Autodesk Inventor part; units mm, degrees
(part 2 of 6)
  line L875 (-91.9006, -60.9474) -> (-91.9173, -60.9168) projected
  line L876 (-91.9173, -60.9168) -> (-91.9334, -60.8858) projected
  line L877 (-91.9334, -60.8858) -> (-91.949, -60.8546) projected
  line L878 (-91.949, -60.8546) -> (-91.964, -60.823) projected
  line L879 (-91.964, -60.823) -> (-91.9785, -60.7913) projected
  line L880 (-91.9785, -60.7913) -> (-91.9924, -60.7593) projected
  line L881 (-91.9924, -60.7593) -> (-92.0058, -60.727) projected
  line L882 (-92.0058, -60.727) -> (-92.0186, -60.6945) projected
  line L883 (-92.0186, -60.6945) -> (-92.0308, -60.6618) projected
  line L884 (-92.0308, -60.6618) -> (-92.0424, -60.6289) projected
  line L885 (-92.0424, -60.6289) -> (-92.0535, -60.5958) projected
  line L886 (-92.0535, -60.5958) -> (-92.064, -60.5626) projected
  line L887 (-92.064, -60.5626) -> (-92.0739, -60.5291) projected
  line L888 (-92.0739, -60.5291) -> (-92.0833, -60.4954) projected
  line L889 (-92.0833, -60.4954) -> (-92.092, -60.4617) projected
  line L890 (-92.092, -60.4617) -> (-92.1001, -60.4277) projected
  line L891 (-92.1001, -60.4277) -> (-92.1077, -60.3936) projected
  line L892 (-92.1077, -60.3936) -> (-92.1147, -60.3594) projected
  line L893 (-92.1147, -60.3594) -> (-92.121, -60.3251) projected
  line L894 (-92.121, -60.3251) -> (-92.1268, -60.2907) projected
  line L895 (-92.1268, -60.2907) -> (-92.1319, -60.2562) projected
  line L896 (-92.1319, -60.2562) -> (-92.1365, -60.2215) projected
  line L897 (-92.1365, -60.2215) -> (-92.1404, -60.1869) projected
  line L898 (-92.1404, -60.1869) -> (-92.1438, -60.1521) projected
  line L899 (-92.1438, -60.1521) -> (-92.1465, -60.1173) projected
  line L900 (-92.1465, -60.1173) -> (-92.1487, -60.0825) projected
  line L901 (-92.1487, -60.0825) -> (-92.1502, -60.0476) projected
  line L902 (-92.1502, -60.0476) -> (-92.1511, -60.0127) projected
  line L903 (-92.1511, -60.0127) -> (-92.1514, -59.9778) projected
  line L904 (-92.1514, -59.9778) -> (-92.1511, -59.9429) projected
  line L905 (-92.1511, -59.9429) -> (-92.1502, -59.908) projected
  line L906 (-92.1502, -59.908) -> (-92.1487, -59.8731) projected
  line L907 (-92.1487, -59.8731) -> (-92.1465, -59.8383) projected
  line L908 (-92.1465, -59.8383) -> (-92.1438, -59.8035) projected
  line L909 (-92.1438, -59.8035) -> (-92.1404, -59.7688) projected
  line L910 (-92.1404, -59.7688) -> (-92.1365, -59.7341) projected
  line L911 (-92.1365, -59.7341) -> (-92.1319, -59.6995) projected
  line L912 (-92.1319, -59.6995) -> (-92.1268, -59.6649) projected
  line L913 (-92.1268, -59.6649) -> (-92.121, -59.6305) projected
  line L914 (-92.121, -59.6305) -> (-92.1147, -59.5962) projected
  line L915 (-92.1147, -59.5962) -> (-92.1077, -59.562) projected
  line L916 (-92.1077, -59.562) -> (-92.1001, -59.5279) projected
  line L917 (-92.1001, -59.5279) -> (-92.092, -59.494) projected
  line L918 (-92.092, -59.494) -> (-92.0833, -59.4602) projected
  line L919 (-92.0833, -59.4602) -> (-92.0739, -59.4265) projected
  line L920 (-92.0739, -59.4265) -> (-92.064, -59.3931) projected
  line L921 (-92.064, -59.3931) -> (-92.0535, -59.3598) projected
  line L922 (-92.0535, -59.3598) -> (-92.0424, -59.3267) projected
  line L923 (-92.0424, -59.3267) -> (-92.0308, -59.2938) projected
  line L924 (-92.0308, -59.2938) -> (-92.0186, -59.2611) projected
  line L925 (-92.0186, -59.2611) -> (-92.0058, -59.2286) projected
  line L926 (-92.0058, -59.2286) -> (-91.9924, -59.1963) projected
  line L927 (-91.9924, -59.1963) -> (-91.9785, -59.1643) projected
  line L928 (-91.9785, -59.1643) -> (-91.964, -59.1326) projected
  line L929 (-91.964, -59.1326) -> (-91.949, -59.1011) projected
  line L930 (-91.949, -59.1011) -> (-91.9334, -59.0698) projected
  line L931 (-91.9334, -59.0698) -> (-91.9173, -59.0389) projected
  line L932 (-91.9173, -59.0389) -> (-91.9006, -59.0082) projected
  line L933 (-91.9006, -59.0082) -> (-91.8835, -58.9778) projected
  line L934 (-91.8835, -58.9778) -> (-91.8657, -58.9477) projected
  line L935 (-91.8657, -58.9477) -> (-91.8475, -58.918) projected
  line L936 (-91.8475, -58.918) -> (-91.8287, -58.8885) projected
  line L937 (-91.8287, -58.8885) -> (-91.8095, -58.8594) projected
  line L938 (-91.8095, -58.8594) -> (-91.7897, -58.8307) projected
  line L939 (-91.7897, -58.8307) -> (-91.7694, -58.8022) projected
  line L940 (-91.7694, -58.8022) -> (-91.7487, -58.7742) projected
  line L941 (-91.7487, -58.7742) -> (-91.7274, -58.7465) projected
  line L942 (-91.7274, -58.7465) -> (-91.7057, -58.7192) projected
  line L943 (-91.7057, -58.7192) -> (-91.6835, -58.6922) projected
  line L944 (-91.6835, -58.6922) -> (-91.6608, -58.6657) projected
  line L945 (-91.6608, -58.6657) -> (-91.6377, -58.6396) projected
  line L946 (-91.6377, -58.6396) -> (-91.6141, -58.6138) projected
  line L947 (-91.6141, -58.6138) -> (-91.5901, -58.5885) projected
  line L948 (-91.5901, -58.5885) -> (-91.5656, -58.5636) projected
  line L949 (-91.5656, -58.5636) -> (-91.5407, -58.5391) projected
  line L950 (-91.5407, -58.5391) -> (-91.5154, -58.5151) projected
  line L951 (-91.5154, -58.5151) -> (-91.4897, -58.4915) projected
  line L952 (-91.4897, -58.4915) -> (-91.4635, -58.4684) projected
  line L953 (-91.4635, -58.4684) -> (-91.437, -58.4457) projected
  line L954 (-91.437, -58.4457) -> (-91.41, -58.4235) projected
  line L955 (-91.41, -58.4235) -> (-91.3827, -58.4018) projected
  line L956 (-91.3827, -58.4018) -> (-91.355, -58.3805) projected
  line L957 (-91.355, -58.3805) -> (-91.327, -58.3598) projected
  line L958 (-91.327, -58.3598) -> (-91.2986, -58.3395) projected
  line L959 (-91.2986, -58.3395) -> (-91.2698, -58.3197) projected
  line L960 (-91.2698, -58.3197) -> (-91.2407, -58.3005) projected
  line L961 (-91.2407, -58.3005) -> (-91.2112, -58.2817) projected
  line L962 (-91.2112, -58.2817) -> (-91.1815, -58.2635) projected
  line L963 (-91.1815, -58.2635) -> (-91.1514, -58.2458) projected
  line L964 (-91.1514, -58.2458) -> (-91.121, -58.2286) projected
  line L965 (-91.121, -58.2286) -> (-91.0904, -58.2119) projected
  line L966 (-91.0904, -58.2119) -> (-91.0594, -58.1958) projected
  line L967 (-91.0594, -58.1958) -> (-91.0282, -58.1802) projected
  line L968 (-91.0282, -58.1802) -> (-90.9966, -58.1652) projected
  line L969 (-90.9966, -58.1652) -> (-90.9649, -58.1507) projected
  line L970 (-90.9649, -58.1507) -> (-90.9329, -58.1368) projected
  line L971 (-90.9329, -58.1368) -> (-90.9006, -58.1234) projected
  line L972 (-90.9006, -58.1234) -> (-90.8681, -58.1107) projected
  line L973 (-90.8681, -58.1107) -> (-90.8354, -58.0984) projected
  line L974 (-90.8354, -58.0984) -> (-90.8025, -58.0868) projected
  line L975 (-90.8025, -58.0868) -> (-90.7694, -58.0757) projected
  line L976 (-90.7694, -58.0757) -> (-90.7362, -58.0652) projected
  line L977 (-90.7362, -58.0652) -> (-90.7027, -58.0553) projected
  line L978 (-90.7027, -58.0553) -> (-90.669, -58.046) projected
  line L979 (-90.669, -58.046) -> (-90.6353, -58.0372) projected
  line L980 (-90.6353, -58.0372) -> (-90.6013, -58.0291) projected
  line L981 (-90.6013, -58.0291) -> (-90.5672, -58.0215) projected
  line L982 (-90.5672, -58.0215) -> (-90.533, -58.0146) projected
  line L983 (-90.533, -58.0146) -> (-90.4987, -58.0082) projected
  line L984 (-90.4987, -58.0082) -> (-90.4643, -58.0024) projected
  line L985 (-90.4643, -58.0024) -> (-90.4298, -57.9973) projected
  line L986 (-90.4298, -57.9973) -> (-90.3951, -57.9927) projected
  line L987 (-90.3951, -57.9927) -> (-90.3605, -57.9888) projected
  line L988 (-90.3605, -57.9888) -> (-90.3257, -57.9854) projected
  line L989 (-90.3257, -57.9854) -> (-90.2909, -57.9827) projected
  line L990 (-90.2909, -57.9827) -> (-90.2561, -57.9806) projected
  line L991 (-90.2561, -57.9806) -> (-90.2212, -57.979) projected
  line L992 (-90.2212, -57.979) -> (-90.1863, -57.9781) projected
  line L993 (-90.1863, -57.9781) -> (-90.1514, -57.9778) projected
  line L994 (-90.1514, -57.9778) -> (-90.1165, -57.9781) projected
  line L995 (-90.1165, -57.9781) -> (-90.0816, -57.979) projected
  line L996 (-90.0816, -57.979) -> (-90.0467, -57.9806) projected
  line L997 (-90.0467, -57.9806) -> (-90.0119, -57.9827) projected
  line L998 (-90.0119, -57.9827) -> (-89.9771, -57.9854) projected
  line L999 (-89.9771, -57.9854) -> (-89.9424, -57.9888) projected
  line L1000 (-89.9424, -57.9888) -> (-89.9077, -57.9927) projected
  line L1001 (-89.9077, -57.9927) -> (-89.8731, -57.9973) projected
  line L1002 (-89.8731, -57.9973) -> (-89.8385, -58.0024) projected
  line L1003 (-89.8385, -58.0024) -> (-89.8041, -58.0082) projected
  line L1004 (-89.8041, -58.0082) -> (-89.7698, -58.0146) projected
  line L1005 (-89.7698, -58.0146) -> (-89.7356, -58.0215) projected
  line L1006 (-89.7356, -58.0215) -> (-89.7015, -58.0291) projected
  line L1007 (-89.7015, -58.0291) -> (-89.6676, -58.0372) projected
  line L1008 (-89.6676, -58.0372) -> (-89.6338, -58.046) projected
  line L1009 (-89.6338, -58.046) -> (-89.6001, -58.0553) projected
  line L1010 (-89.6001, -58.0553) -> (-89.5667, -58.0652) projected
  line L1011 (-89.5667, -58.0652) -> (-89.5334, -58.0757) projected
  line L1012 (-89.5334, -58.0757) -> (-89.5003, -58.0868) projected
  line L1013 (-89.5003, -58.0868) -> (-89.4674, -58.0984) projected
  line L1014 (-89.4674, -58.0984) -> (-89.4347, -58.1107) projected
  line L1015 (-89.4347, -58.1107) -> (-89.4022, -58.1234) projected
  line L1016 (-89.4022, -58.1234) -> (-89.3699, -58.1368) projected
  line L1017 (-89.3699, -58.1368) -> (-89.3379, -58.1507) projected
  line L1018 (-89.3379, -58.1507) -> (-89.3062, -58.1652) projected
  line L1019 (-89.3062, -58.1652) -> (-89.2747, -58.1802) projected
  line L1020 (-89.2747, -58.1802) -> (-89.2434, -58.1958) projected
  line L1021 (-89.2434, -58.1958) -> (-89.2125, -58.2119) projected
  line L1022 (-89.2125, -58.2119) -> (-89.1818, -58.2286) projected
  line L1023 (-89.1818, -58.2286) -> (-89.1514, -58.2458) projected
  line L1024 (-89.1514, -58.2458) -> (-89.1213, -58.2635) projected
  line L1025 (-89.1213, -58.2635) -> (-89.0916, -58.2817) projected
  line L1026 (-89.0916, -58.2817) -> (-89.0621, -58.3005) projected
  line L1027 (-89.0621, -58.3005) -> (-89.033, -58.3197) projected
  line L1028 (-89.033, -58.3197) -> (-89.0043, -58.3395) projected
  line L1029 (-89.0043, -58.3395) -> (-88.9758, -58.3598) projected
  line L1030 (-88.9758, -58.3598) -> (-88.9478, -58.3805) projected
  line L1031 (-88.9478, -58.3805) -> (-88.9201, -58.4018) projected
  line L1032 (-88.9201, -58.4018) -> (-88.8928, -58.4235) projected
  line L1033 (-88.8928, -58.4235) -> (-88.8658, -58.4457) projected
  line L1034 (-88.8658, -58.4457) -> (-88.8393, -58.4684) projected
  line L1035 (-88.8393, -58.4684) -> (-88.8132, -58.4915) projected
  line L1036 (-88.8132, -58.4915) -> (-88.7874, -58.5151) projected
  line L1037 (-88.7874, -58.5151) -> (-88.7621, -58.5391) projected
  line L1038 (-88.7621, -58.5391) -> (-88.7372, -58.5636) projected
  line L1039 (-88.7372, -58.5636) -> (-88.7127, -58.5885) projected
  line L1040 (-88.7127, -58.5885) -> (-88.6887, -58.6138) projected
  line L1041 (-88.6887, -58.6138) -> (-88.6651, -58.6396) projected
  line L1042 (-88.6651, -58.6396) -> (-88.642, -58.6657) projected
  line L1043 (-88.642, -58.6657) -> (-88.6193, -58.6922) projected
  line L1044 (-88.6193, -58.6922) -> (-88.5971, -58.7192) projected
  line L1045 (-88.5971, -58.7192) -> (-88.5754, -58.7465) projected
  line L1046 (-88.5754, -58.7465) -> (-88.5541, -58.7742) projected
  line L1047 (-88.5541, -58.7742) -> (-88.5334, -58.8022) projected
  line L1048 (-88.5334, -58.8022) -> (-88.5131, -58.8307) projected
  line L1049 (-88.5131, -58.8307) -> (-88.4933, -58.8594) projected
  line L1050 (-88.4933, -58.8594) -> (-88.4741, -58.8885) projected
  line L1051 (-88.4741, -58.8885) -> (-88.4553, -58.918) projected
  line L1052 (-88.4553, -58.918) -> (-88.4371, -58.9477) projected
  line L1053 (-88.4371, -58.9477) -> (-88.4194, -58.9778) projected
  line L1054 (-88.4194, -58.9778) -> (-88.4022, -59.0082) projected
  line L1055 (-88.4022, -59.0082) -> (-88.3855, -59.0389) projected
  line L1056 (-88.3855, -59.0389) -> (-88.3694, -59.0698) projected
  line L1057 (-88.3694, -59.0698) -> (-88.3538, -59.1011) projected
  line L1058 (-88.3538, -59.1011) -> (-88.3388, -59.1326) projected
  line L1059 (-88.3388, -59.1326) -> (-88.3243, -59.1643) projected
  line L1060 (-88.3243, -59.1643) -> (-88.3104, -59.1963) projected
  line L1061 (-88.3104, -59.1963) -> (-88.297, -59.2286) projected
  line L1062 (-88.297, -59.2286) -> (-88.2843, -59.2611) projected
  line L1063 (-88.2843, -59.2611) -> (-88.272, -59.2938) projected
  line L1064 (-88.272, -59.2938) -> (-88.2604, -59.3267) projected
  line L1065 (-88.2604, -59.3267) -> (-88.2493, -59.3598) projected
  line L1066 (-88.2493, -59.3598) -> (-88.2388, -59.3931) projected
  line L1067 (-88.2388, -59.3931) -> (-88.2289, -59.4265) projected
  line L1068 (-88.2289, -59.4265) -> (-88.2196, -59.4602) projected
  line L1069 (-88.2196, -59.4602) -> (-88.2108, -59.494) projected
  line L1070 (-88.2108, -59.494) -> (-88.2027, -59.5279) projected
  line L1071 (-88.2027, -59.5279) -> (-88.1951, -59.562) projected
  line L1072 (-88.1951, -59.562) -> (-88.1882, -59.5962) projected
  line L1073 (-88.1882, -59.5962) -> (-88.1818, -59.6305) projected
  line L1074 (-88.1818, -59.6305) -> (-88.176, -59.6649) projected
  line L1075 (-88.176, -59.6649) -> (-88.1709, -59.6995) projected
  line L1076 (-88.1709, -59.6995) -> (-88.1663, -59.7341) projected
  line L1077 (-88.1663, -59.7341) -> (-88.1624, -59.7688) projected
  line L1078 (-88.1624, -59.7688) -> (-88.159, -59.8035) projected
  line L1079 (-88.159, -59.8035) -> (-88.1563, -59.8383) projected
  line L1080 (-88.1563, -59.8383) -> (-88.1542, -59.8731) projected
  line L1081 (-88.1542, -59.8731) -> (-88.1526, -59.908) projected
  line L1082 (-88.1526, -59.908) -> (-88.1517, -59.9429) projected
  line L1083 (-88.1517, -59.9429) -> (-88.1514, -59.9778) projected
  line L1084 (-88.1563, 60.1617) -> (-88.1542, 60.1269) projected
  line L1085 (-88.1542, 60.1269) -> (-88.1526, 60.092) projected
  line L1086 (-88.1526, 60.092) -> (-88.1517, 60.0571) projected
  line L1087 (-88.1517, 60.0571) -> (-88.1514, 60.0222) projected
  line L1088 (-88.1514, 60.0222) -> (-88.1517, 59.9873) projected
  line L1089 (-88.1517, 59.9873) -> (-88.1526, 59.9524) projected
  line L1090 (-88.1526, 59.9524) -> (-88.1542, 59.9175) projected
  line L1091 (-88.1542, 59.9175) -> (-88.1563, 59.8827) projected
  line L1092 (-88.1563, 59.8827) -> (-88.159, 59.8479) projected
  line L1093 (-88.159, 59.8479) -> (-88.1624, 59.8131) projected
  line L1094 (-88.1624, 59.8131) -> (-88.1663, 59.7785) projected
  line L1095 (-88.1663, 59.7785) -> (-88.1709, 59.7439) projected
  line L1096 (-88.1709, 59.7439) -> (-88.176, 59.7093) projected
  line L1097 (-88.176, 59.7093) -> (-88.1818, 59.6749) projected
  line L1098 (-88.1818, 59.6749) -> (-88.1882, 59.6406) projected
  line L1099 (-88.1882, 59.6406) -> (-88.1951, 59.6064) projected
  line L1100 (-88.1951, 59.6064) -> (-88.2027, 59.5723) projected
  line L1101 (-88.2027, 59.5723) -> (-88.2108, 59.5384) projected
  line L1102 (-88.2108, 59.5384) -> (-88.2196, 59.5046) projected
  line L1103 (-88.2196, 59.5046) -> (-88.2289, 59.4709) projected
  line L1104 (-88.2289, 59.4709) -> (-88.2388, 59.4375) projected
  line L1105 (-88.2388, 59.4375) -> (-88.2493, 59.4042) projected
  line L1106 (-88.2493, 59.4042) -> (-88.2604, 59.3711) projected
  line L1107 (-88.2604, 59.3711) -> (-88.272, 59.3382) projected
  line L1108 (-88.272, 59.3382) -> (-88.2843, 59.3055) projected
  line L1109 (-88.2843, 59.3055) -> (-88.297, 59.273) projected
  line L1110 (-88.297, 59.273) -> (-88.3104, 59.2407) projected
  line L1111 (-88.3104, 59.2407) -> (-88.3243, 59.2087) projected
  line L1112 (-88.3243, 59.2087) -> (-88.3388, 59.177) projected
  line L1113 (-88.3388, 59.177) -> (-88.3538, 59.1455) projected
  line L1114 (-88.3538, 59.1455) -> (-88.3694, 59.1142) projected
  line L1115 (-88.3694, 59.1142) -> (-88.3855, 59.0833) projected
  line L1116 (-88.3855, 59.0833) -> (-88.4022, 59.0526) projected
  line L1117 (-88.4022, 59.0526) -> (-88.4194, 59.0222) projected
  line L1118 (-88.4194, 59.0222) -> (-88.4371, 58.9921) projected
  line L1119 (-88.4371, 58.9921) -> (-88.4553, 58.9624) projected
  line L1120 (-88.4553, 58.9624) -> (-88.4741, 58.9329) projected
  line L1121 (-88.4741, 58.9329) -> (-88.4933, 58.9038) projected
  line L1122 (-88.4933, 58.9038) -> (-88.5131, 58.8751) projected
  line L1123 (-88.5131, 58.8751) -> (-88.5334, 58.8466) projected
  line L1124 (-88.5334, 58.8466) -> (-88.5541, 58.8186) projected
  line L1125 (-88.5541, 58.8186) -> (-88.5754, 58.7909) projected
  line L1126 (-88.5754, 58.7909) -> (-88.5971, 58.7636) projected
  line L1127 (-88.5971, 58.7636) -> (-88.6193, 58.7366) projected
  line L1128 (-88.6193, 58.7366) -> (-88.642, 58.7101) projected
  line L1129 (-88.642, 58.7101) -> (-88.6651, 58.6839) projected
  line L1130 (-88.6651, 58.6839) -> (-88.6887, 58.6582) projected
  line L1131 (-88.6887, 58.6582) -> (-88.7127, 58.6329) projected
  line L1132 (-88.7127, 58.6329) -> (-88.7372, 58.608) projected
  line L1133 (-88.7372, 58.608) -> (-88.7621, 58.5835) projected
  line L1134 (-88.7621, 58.5835) -> (-88.7874, 58.5595) projected
  line L1135 (-88.7874, 58.5595) -> (-88.8132, 58.5359) projected
  line L1136 (-88.8132, 58.5359) -> (-88.8393, 58.5128) projected
  line L1137 (-88.8393, 58.5128) -> (-88.8658, 58.4901) projected
  line L1138 (-88.8658, 58.4901) -> (-88.8928, 58.4679) projected
  line L1139 (-88.8928, 58.4679) -> (-88.9201, 58.4462) projected
  line L1140 (-88.9201, 58.4462) -> (-88.9478, 58.4249) projected
  line L1141 (-88.9478, 58.4249) -> (-88.9758, 58.4042) projected
  line L1142 (-88.9758, 58.4042) -> (-89.0043, 58.3839) projected
  line L1143 (-89.0043, 58.3839) -> (-89.033, 58.3641) projected
  line L1144 (-89.033, 58.3641) -> (-89.0621, 58.3449) projected
  line L1145 (-89.0621, 58.3449) -> (-89.0916, 58.3261) projected
  line L1146 (-89.0916, 58.3261) -> (-89.1213, 58.3079) projected
  line L1147 (-89.1213, 58.3079) -> (-89.1514, 58.2902) projected
  line L1148 (-89.1514, 58.2902) -> (-89.1818, 58.273) projected
  line L1149 (-89.1818, 58.273) -> (-89.2125, 58.2563) projected
  line L1150 (-89.2125, 58.2563) -> (-89.2434, 58.2402) projected
  line L1151 (-89.2434, 58.2402) -> (-89.2747, 58.2246) projected
  line L1152 (-89.2747, 58.2246) -> (-89.3062, 58.2096) projected
  line L1153 (-89.3062, 58.2096) -> (-89.3379, 58.1951) projected
  line L1154 (-89.3379, 58.1951) -> (-89.3699, 58.1812) projected
  line L1155 (-89.3699, 58.1812) -> (-89.4022, 58.1678) projected
  line L1156 (-89.4022, 58.1678) -> (-89.4347, 58.155) projected
  line L1157 (-89.4347, 58.155) -> (-89.4674, 58.1428) projected
  line L1158 (-89.4674, 58.1428) -> (-89.5003, 58.1312) projected
  line L1159 (-89.5003, 58.1312) -> (-89.5334, 58.1201) projected
  line L1160 (-89.5334, 58.1201) -> (-89.5667, 58.1096) projected
  line L1161 (-89.5667, 58.1096) -> (-89.6001, 58.0997) projected
  line L1162 (-89.6001, 58.0997) -> (-89.6338, 58.0904) projected
  line L1163 (-89.6338, 58.0904) -> (-89.6676, 58.0816) projected
  line L1164 (-89.6676, 58.0816) -> (-89.7015, 58.0735) projected
  line L1165 (-89.7015, 58.0735) -> (-89.7356, 58.0659) projected
  line L1166 (-89.7356, 58.0659) -> (-89.7698, 58.059) projected
  line L1167 (-89.7698, 58.059) -> (-89.8041, 58.0526) projected
  line L1168 (-89.8041, 58.0526) -> (-89.8385, 58.0468) projected
  line L1169 (-89.8385, 58.0468) -> (-89.8731, 58.0417) projected
  line L1170 (-89.8731, 58.0417) -> (-89.9077, 58.0371) projected
  line L1171 (-89.9077, 58.0371) -> (-89.9424, 58.0332) projected
  line L1172 (-89.9424, 58.0332) -> (-89.9771, 58.0298) projected
  line L1173 (-89.9771, 58.0298) -> (-90.0119, 58.0271) projected
  line L1174 (-90.0119, 58.0271) -> (-90.0467, 58.0249) projected
  line L1175 (-90.0467, 58.0249) -> (-90.0816, 58.0234) projected
  line L1176 (-90.0816, 58.0234) -> (-90.1165, 58.0225) projected
  line L1177 (-90.1165, 58.0225) -> (-90.1514, 58.0222) projected
  line L1178 (-90.1514, 58.0222) -> (-90.1863, 58.0225) projected
  line L1179 (-90.1863, 58.0225) -> (-90.2212, 58.0234) projected
  line L1180 (-90.2212, 58.0234) -> (-90.2561, 58.0249) projected
  line L1181 (-90.2561, 58.0249) -> (-90.2909, 58.0271) projected
  line L1182 (-90.2909, 58.0271) -> (-90.3257, 58.0298) projected
  line L1183 (-90.3257, 58.0298) -> (-90.3605, 58.0332) projected
  line L1184 (-90.3605, 58.0332) -> (-90.3951, 58.0371) projected
  line L1185 (-90.3951, 58.0371) -> (-90.4298, 58.0417) projected
  line L1186 (-90.4298, 58.0417) -> (-90.4643, 58.0468) projected
  line L1187 (-90.4643, 58.0468) -> (-90.4987, 58.0526) projected
  line L1188 (-90.4987, 58.0526) -> (-90.533, 58.059) projected
  line L1189 (-90.533, 58.059) -> (-90.5672, 58.0659) projected
  line L1190 (-90.5672, 58.0659) -> (-90.6013, 58.0735) projected
  line L1191 (-90.6013, 58.0735) -> (-90.6353, 58.0816) projected
  line L1192 (-90.6353, 58.0816) -> (-90.669, 58.0904) projected
  line L1193 (-90.669, 58.0904) -> (-90.7027, 58.0997) projected
  line L1194 (-90.7027, 58.0997) -> (-90.7362, 58.1096) projected
  line L1195 (-90.7362, 58.1096) -> (-90.7694, 58.1201) projected
  line L1196 (-90.7694, 58.1201) -> (-90.8025, 58.1312) projected
  line L1197 (-90.8025, 58.1312) -> (-90.8354, 58.1428) projected
  line L1198 (-90.8354, 58.1428) -> (-90.8681, 58.155) projected
  line L1199 (-90.8681, 58.155) -> (-90.9006, 58.1678) projected
  line L1200 (-90.9006, 58.1678) -> (-90.9329, 58.1812) projected
  line L1201 (-90.9329, 58.1812) -> (-90.9649, 58.1951) projected
  line L1202 (-90.9649, 58.1951) -> (-90.9966, 58.2096) projected
  line L1203 (-90.9966, 58.2096) -> (-91.0282, 58.2246) projected
  line L1204 (-91.0282, 58.2246) -> (-91.0594, 58.2402) projected
  line L1205 (-91.0594, 58.2402) -> (-91.0904, 58.2563) projected
  line L1206 (-91.0904, 58.2563) -> (-91.121, 58.273) projected
  line L1207 (-91.121, 58.273) -> (-91.1514, 58.2902) projected
  line L1208 (-91.1514, 58.2902) -> (-91.1815, 58.3079) projected
  line L1209 (-91.1815, 58.3079) -> (-91.2112, 58.3261) projected
  line L1210 (-91.2112, 58.3261) -> (-91.2407, 58.3449) projected
  line L1211 (-91.2407, 58.3449) -> (-91.2698, 58.3641) projected
  line L1212 (-91.2698, 58.3641) -> (-91.2986, 58.3839) projected
  line L1213 (-91.2986, 58.3839) -> (-91.327, 58.4042) projected
  line L1214 (-91.327, 58.4042) -> (-91.355, 58.4249) projected
  line L1215 (-91.355, 58.4249) -> (-91.3827, 58.4462) projected
  line L1216 (-91.3827, 58.4462) -> (-91.41, 58.4679) projected
  line L1217 (-91.41, 58.4679) -> (-91.437, 58.4901) projected
  line L1218 (-91.437, 58.4901) -> (-91.4635, 58.5128) projected
  line L1219 (-91.4635, 58.5128) -> (-91.4897, 58.5359) projected
  line L1220 (-91.4897, 58.5359) -> (-91.5154, 58.5595) projected
  line L1221 (-91.5154, 58.5595) -> (-91.5407, 58.5835) projected
  line L1222 (-91.5407, 58.5835) -> (-91.5656, 58.608) projected
  line L1223 (-91.5656, 58.608) -> (-91.5901, 58.6329) projected
  line L1224 (-91.5901, 58.6329) -> (-91.6141, 58.6582) projected
  line L1225 (-91.6141, 58.6582) -> (-91.6377, 58.6839) projected
  line L1226 (-91.6377, 58.6839) -> (-91.6608, 58.7101) projected
  line L1227 (-91.6608, 58.7101) -> (-91.6835, 58.7366) projected
  line L1228 (-91.6835, 58.7366) -> (-91.7057, 58.7636) projected
  line L1229 (-91.7057, 58.7636) -> (-91.7274, 58.7909) projected
  line L1230 (-91.7274, 58.7909) -> (-91.7487, 58.8186) projected
  line L1231 (-91.7487, 58.8186) -> (-91.7694, 58.8466) projected
  line L1232 (-91.7694, 58.8466) -> (-91.7897, 58.8751) projected
  line L1233 (-91.7897, 58.8751) -> (-91.8095, 58.9038) projected
  line L1234 (-91.8095, 58.9038) -> (-91.8287, 58.9329) projected
  line L1235 (-91.8287, 58.9329) -> (-91.8475, 58.9624) projected
  line L1236 (-91.8475, 58.9624) -> (-91.8657, 58.9921) projected
  line L1237 (-91.8657, 58.9921) -> (-91.8835, 59.0222) projected
  line L1238 (-91.8835, 59.0222) -> (-91.9006, 59.0526) projected
  line L1239 (-91.9006, 59.0526) -> (-91.9173, 59.0833) projected
  line L1240 (-91.9173, 59.0833) -> (-91.9334, 59.1142) projected
  line L1241 (-91.9334, 59.1142) -> (-91.949, 59.1455) projected
  line L1242 (-91.949, 59.1455) -> (-91.964, 59.177) projected
  line L1243 (-91.964, 59.177) -> (-91.9785, 59.2087) projected
  line L1244 (-91.9785, 59.2087) -> (-91.9924, 59.2407) projected
  line L1245 (-91.9924, 59.2407) -> (-92.0058, 59.273) projected
  line L1246 (-92.0058, 59.273) -> (-92.0186, 59.3055) projected
  line L1247 (-92.0186, 59.3055) -> (-92.0308, 59.3382) projected
  line L1248 (-92.0308, 59.3382) -> (-92.0424, 59.3711) projected
  line L1249 (-92.0424, 59.3711) -> (-92.0535, 59.4042) projected
  line L1250 (-92.0535, 59.4042) -> (-92.064, 59.4375) projected
  line L1251 (-92.064, 59.4375) -> (-92.0739, 59.4709) projected
  line L1252 (-92.0739, 59.4709) -> (-92.0833, 59.5046) projected
  line L1253 (-92.0833, 59.5046) -> (-92.092, 59.5384) projected
  line L1254 (-92.092, 59.5384) -> (-92.1001, 59.5723) projected
  line L1255 (-92.1001, 59.5723) -> (-92.1077, 59.6064) projected
  line L1256 (-92.1077, 59.6064) -> (-92.1147, 59.6406) projected
  line L1257 (-92.1147, 59.6406) -> (-92.121, 59.6749) projected
  line L1258 (-92.121, 59.6749) -> (-92.1268, 59.7093) projected
  line L1259 (-92.1268, 59.7093) -> (-92.1319, 59.7439) projected
  line L1260 (-92.1319, 59.7439) -> (-92.1365, 59.7785) projected
  line L1261 (-92.1365, 59.7785) -> (-92.1404, 59.8131) projected
  line L1262 (-92.1404, 59.8131) -> (-92.1438, 59.8479) projected
  line L1263 (-92.1438, 59.8479) -> (-92.1465, 59.8827) projected
  line L1264 (-92.1465, 59.8827) -> (-92.1487, 59.9175) projected
  line L1265 (-92.1487, 59.9175) -> (-92.1502, 59.9524) projected
  line L1266 (-92.1502, 59.9524) -> (-92.1511, 59.9873) projected
  line L1267 (-92.1511, 59.9873) -> (-92.1514, 60.0222) projected
  line L1268 (-92.1514, 60.0222) -> (-92.1511, 60.0571) projected
  line L1269 (-92.1511, 60.0571) -> (-92.1502, 60.092) projected
  line L1270 (-92.1502, 60.092) -> (-92.1487, 60.1269) projected
  line L1271 (-92.1487, 60.1269) -> (-92.1465, 60.1617) projected
  line L1272 (-92.1465, 60.1617) -> (-92.1438, 60.1965) projected
  line L1273 (-92.1438, 60.1965) -> (-92.1404, 60.2313) projected
  line L1274 (-92.1404, 60.2313) -> (-92.1365, 60.2659) projected
  line L1275 (-92.1365, 60.2659) -> (-92.1319, 60.3005) projected
  line L1276 (-92.1319, 60.3005) -> (-92.1268, 60.3351) projected
  line L1277 (-92.1268, 60.3351) -> (-92.121, 60.3695) projected
  line L1278 (-92.121, 60.3695) -> (-92.1147, 60.4038) projected
  line L1279 (-92.1147, 60.4038) -> (-92.1077, 60.438) projected
  line L1280 (-92.1077, 60.438) -> (-92.1001, 60.4721) projected
  line L1281 (-92.1001, 60.4721) -> (-92.092, 60.506) projected
  line L1282 (-92.092, 60.506) -> (-92.0833, 60.5398) projected
  line L1283 (-92.0833, 60.5398) -> (-92.0739, 60.5735) projected
  line L1284 (-92.0739, 60.5735) -> (-92.064, 60.6069) projected
  line L1285 (-92.064, 60.6069) -> (-92.0535, 60.6402) projected
  line L1286 (-92.0535, 60.6402) -> (-92.0424, 60.6733) projected
  line L1287 (-92.0424, 60.6733) -> (-92.0308, 60.7062) projected
  line L1288 (-92.0308, 60.7062) -> (-92.0186, 60.7389) projected
  line L1289 (-92.0186, 60.7389) -> (-92.0058, 60.7714) projected
  line L1290 (-92.0058, 60.7714) -> (-91.9924, 60.8037) projected
  line L1291 (-91.9924, 60.8037) -> (-91.9785, 60.8357) projected
  line L1292 (-91.9785, 60.8357) -> (-91.964, 60.8674) projected
  line L1293 (-91.964, 60.8674) -> (-91.949, 60.8989) projected
  line L1294 (-91.949, 60.8989) -> (-91.9334, 60.9302) projected
  line L1295 (-91.9334, 60.9302) -> (-91.9173, 60.9611) projected
  line L1296 (-91.9173, 60.9611) -> (-91.9006, 60.9918) projected
  line L1297 (-91.9006, 60.9918) -> (-91.8835, 61.0222) projected
  line L1298 (-91.8835, 61.0222) -> (-91.8657, 61.0523) projected
  line L1299 (-91.8657, 61.0523) -> (-91.8475, 61.082) projected
  line L1300 (-91.8475, 61.082) -> (-91.8287, 61.1115) projected
  line L1301 (-91.8287, 61.1115) -> (-91.8095, 61.1406) projected
  line L1302 (-91.8095, 61.1406) -> (-91.7897, 61.1694) projected
  line L1303 (-91.7897, 61.1694) -> (-91.7694, 61.1978) projected
  line L1304 (-91.7694, 61.1978) -> (-91.7487, 61.2258) projected
  line L1305 (-91.7487, 61.2258) -> (-91.7274, 61.2535) projected
  line L1306 (-91.7274, 61.2535) -> (-91.7057, 61.2808) projected
  line L1307 (-91.7057, 61.2808) -> (-91.6835, 61.3078) projected
  line L1308 (-91.6835, 61.3078) -> (-91.6608, 61.3343) projected
  line L1309 (-91.6608, 61.3343) -> (-91.6377, 61.3605) projected
  line L1310 (-91.6377, 61.3605) -> (-91.6141, 61.3862) projected
  line L1311 (-91.6141, 61.3862) -> (-91.5901, 61.4115) projected
  line L1312 (-91.5901, 61.4115) -> (-91.5656, 61.4364) projected
  line L1313 (-91.5656, 61.4364) -> (-91.5407, 61.4609) projected
  line L1314 (-91.5407, 61.4609) -> (-91.5154, 61.4849) projected
  line L1315 (-91.5154, 61.4849) -> (-91.4897, 61.5085) projected
  line L1316 (-91.4897, 61.5085) -> (-91.4635, 61.5316) projected
  line L1317 (-91.4635, 61.5316) -> (-91.437, 61.5543) projected
  line L1318 (-91.437, 61.5543) -> (-91.41, 61.5765) projected
  line L1319 (-91.41, 61.5765) -> (-91.3827, 61.5982) projected
  line L1320 (-91.3827, 61.5982) -> (-91.355, 61.6195) projected
  line L1321 (-91.355, 61.6195) -> (-91.327, 61.6402) projected
  line L1322 (-91.327, 61.6402) -> (-91.2986, 61.6605) projected
  line L1323 (-91.2986, 61.6605) -> (-91.2698, 61.6803) projected
  line L1324 (-91.2698, 61.6803) -> (-91.2407, 61.6995) projected
  line L1325 (-91.2407, 61.6995) -> (-91.2112, 61.7183) projected
  line L1326 (-91.2112, 61.7183) -> (-91.1815, 61.7365) projected
  line L1327 (-91.1815, 61.7365) -> (-91.1514, 61.7543) projected
  line L1328 (-91.1514, 61.7543) -> (-91.121, 61.7714) projected
  line L1329 (-91.121, 61.7714) -> (-91.0904, 61.7881) projected
  line L1330 (-91.0904, 61.7881) -> (-91.0594, 61.8042) projected
  line L1331 (-91.0594, 61.8042) -> (-91.0282, 61.8198) projected
  line L1332 (-91.0282, 61.8198) -> (-90.9966, 61.8348) projected
  line L1333 (-90.9966, 61.8348) -> (-90.9649, 61.8493) projected
  line L1334 (-90.9649, 61.8493) -> (-90.9329, 61.8632) projected
  line L1335 (-90.9329, 61.8632) -> (-90.9006, 61.8766) projected
  line L1336 (-90.9006, 61.8766) -> (-90.8681, 61.8894) projected
  line L1337 (-90.8681, 61.8894) -> (-90.8354, 61.9016) projected
  line L1338 (-90.8354, 61.9016) -> (-90.8025, 61.9132) projected
  line L1339 (-90.8025, 61.9132) -> (-90.7694, 61.9243) projected
  line L1340 (-90.7694, 61.9243) -> (-90.7362, 61.9348) projected
  line L1341 (-90.7362, 61.9348) -> (-90.7027, 61.9447) projected
  line L1342 (-90.7027, 61.9447) -> (-90.669, 61.9541) projected
  line L1343 (-90.669, 61.9541) -> (-90.6353, 61.9628) projected
  line L1344 (-90.6353, 61.9628) -> (-90.6013, 61.9709) projected
  line L1345 (-90.6013, 61.9709) -> (-90.5672, 61.9785) projected
  line L1346 (-90.5672, 61.9785) -> (-90.533, 61.9855) projected
  line L1347 (-90.533, 61.9855) -> (-90.4987, 61.9918) projected
  line L1348 (-90.4987, 61.9918) -> (-90.4643, 61.9976) projected
  line L1349 (-90.4643, 61.9976) -> (-90.4298, 62.0027) projected
  line L1350 (-90.4298, 62.0027) -> (-90.3951, 62.0073) projected
  line L1351 (-90.3951, 62.0073) -> (-90.3605, 62.0112) projected
  line L1352 (-90.3605, 62.0112) -> (-90.3257, 62.0146) projected
  line L1353 (-90.3257, 62.0146) -> (-90.2909, 62.0173) projected
  line L1354 (-90.2909, 62.0173) -> (-90.2561, 62.0195) projected
  line L1355 (-90.2561, 62.0195) -> (-90.2212, 62.021) projected
  line L1356 (-90.2212, 62.021) -> (-90.1863, 62.0219) projected
  line L1357 (-90.1863, 62.0219) -> (-90.1514, 62.0222) projected
  line L1358 (-90.1514, 62.0222) -> (-90.1165, 62.0219) projected
  line L1359 (-90.1165, 62.0219) -> (-90.0816, 62.021) projected
  line L1360 (-90.0816, 62.021) -> (-90.0467, 62.0195) projected
  line L1361 (-90.0467, 62.0195) -> (-90.0119, 62.0173) projected
  line L1362 (-90.0119, 62.0173) -> (-89.9771, 62.0146) projected
  line L1363 (-89.9771, 62.0146) -> (-89.9424, 62.0112) projected
  line L1364 (-89.9424, 62.0112) -> (-89.9077, 62.0073) projected
  line L1365 (-89.9077, 62.0073) -> (-89.8731, 62.0027) projected
  line L1366 (-89.8731, 62.0027) -> (-89.8385, 61.9976) projected
  line L1367 (-89.8385, 61.9976) -> (-89.8041, 61.9918) projected
  line L1368 (-89.8041, 61.9918) -> (-89.7698, 61.9855) projected
  line L1369 (-89.7698, 61.9855) -> (-89.7356, 61.9785) projected
  line L1370 (-89.7356, 61.9785) -> (-89.7015, 61.9709) projected
  line L1371 (-89.7015, 61.9709) -> (-89.6676, 61.9628) projected
  line L1372 (-89.6676, 61.9628) -> (-89.6338, 61.9541) projected
  line L1373 (-89.6338, 61.9541) -> (-89.6001, 61.9447) projected
  line L1374 (-89.6001, 61.9447) -> (-89.5667, 61.9348) projected
  line L1375 (-89.5667, 61.9348) -> (-89.5334, 61.9243) projected
  line L1376 (-89.5334, 61.9243) -> (-89.5003, 61.9132) projected
  line L1377 (-89.5003, 61.9132) -> (-89.4674, 61.9016) projected
  line L1378 (-89.4674, 61.9016) -> (-89.4347, 61.8894) projected
  line L1379 (-89.4347, 61.8894) -> (-89.4022, 61.8766) projected
  line L1380 (-89.4022, 61.8766) -> (-89.3699, 61.8632) projected
  line L1381 (-89.3699, 61.8632) -> (-89.3379, 61.8493) projected
  line L1382 (-89.3379, 61.8493) -> (-89.3062, 61.8348) projected
  line L1383 (-89.3062, 61.8348) -> (-89.2747, 61.8198) projected
  line L1384 (-89.2747, 61.8198) -> (-89.2434, 61.8042) projected
  line L1385 (-89.2434, 61.8042) -> (-89.2125, 61.7881) projected
  line L1386 (-89.2125, 61.7881) -> (-89.1818, 61.7714) projected
  line L1387 (-89.1818, 61.7714) -> (-89.1514, 61.7543) projected
  line L1388 (-89.1514, 61.7543) -> (-89.1213, 61.7365) projected
  line L1389 (-89.1213, 61.7365) -> (-89.0916, 61.7183) projected
  line L1390 (-89.0916, 61.7183) -> (-89.0621, 61.6995) projected
  line L1391 (-89.0621, 61.6995) -> (-89.033, 61.6803) projected
  line L1392 (-89.033, 61.6803) -> (-89.0043, 61.6605) projected
  line L1393 (-89.0043, 61.6605) -> (-88.9758, 61.6402) projected
  line L1394 (-88.9758, 61.6402) -> (-88.9478, 61.6195) projected
  line L1395 (-88.9478, 61.6195) -> (-88.9201, 61.5982) projected
  line L1396 (-88.9201, 61.5982) -> (-88.8928, 61.5765) projected
  line L1397 (-88.8928, 61.5765) -> (-88.8658, 61.5543) projected
  line L1398 (-88.8658, 61.5543) -> (-88.8393, 61.5316) projected
  line L1399 (-88.8393, 61.5316) -> (-88.8132, 61.5085) projected
  line L1400 (-88.8132, 61.5085) -> (-88.7874, 61.4849) projected
  line L1401 (-88.7874, 61.4849) -> (-88.7621, 61.4609) projected
  line L1402 (-88.7621, 61.4609) -> (-88.7372, 61.4364) projected
  line L1403 (-88.7372, 61.4364) -> (-88.7127, 61.4115) projected
  line L1404 (-88.7127, 61.4115) -> (-88.6887, 61.3862) projected
  line L1405 (-88.6887, 61.3862) -> (-88.6651, 61.3605) projected
  line L1406 (-88.6651, 61.3605) -> (-88.642, 61.3343) projected
  line L1407 (-88.642, 61.3343) -> (-88.6193, 61.3078) projected
  line L1408 (-88.6193, 61.3078) -> (-88.5971, 61.2808) projected
  line L1409 (-88.5971, 61.2808) -> (-88.5754, 61.2535) projected
  line L1410 (-88.5754, 61.2535) -> (-88.5541, 61.2258) projected
  line L1411 (-88.5541, 61.2258) -> (-88.5334, 61.1978) projected
  line L1412 (-88.5334, 61.1978) -> (-88.5131, 61.1694) projected
  line L1413 (-88.5131, 61.1694) -> (-88.4933, 61.1406) projected
  line L1414 (-88.4933, 61.1406) -> (-88.4741, 61.1115) projected
  line L1415 (-88.4741, 61.1115) -> (-88.4553, 61.082) projected
  line L1416 (-88.4553, 61.082) -> (-88.4371, 61.0523) projected
  line L1417 (-88.4371, 61.0523) -> (-88.4194, 61.0222) projected
  line L1418 (-88.4194, 61.0222) -> (-88.4022, 60.9918) projected
  line L1419 (-88.4022, 60.9918) -> (-88.3855, 60.9611) projected
  line L1420 (-88.3855, 60.9611) -> (-88.3694, 60.9302) projected
  line L1421 (-88.3694, 60.9302) -> (-88.3538, 60.8989) projected
  line L1422 (-88.3538, 60.8989) -> (-88.3388, 60.8674) projected
  line L1423 (-88.3388, 60.8674) -> (-88.3243, 60.8357) projected
  line L1424 (-88.3243, 60.8357) -> (-88.3104, 60.8037) projected
  line L1425 (-88.3104, 60.8037) -> (-88.297, 60.7714) projected
  line L1426 (-88.297, 60.7714) -> (-88.2843, 60.7389) projected
  line L1427 (-88.2843, 60.7389) -> (-88.272, 60.7062) projected
  line L1428 (-88.272, 60.7062) -> (-88.2604, 60.6733) projected
  line L1429 (-88.2604, 60.6733) -> (-88.2493, 60.6402) projected
  line L1430 (-88.2493, 60.6402) -> (-88.2388, 60.6069) projected
  line L1431 (-88.2388, 60.6069) -> (-88.2289, 60.5735) projected
  line L1432 (-88.2289, 60.5735) -> (-88.2196, 60.5398) projected
  line L1433 (-88.2196, 60.5398) -> (-88.2108, 60.506) projected
  line L1434 (-88.2108, 60.506) -> (-88.2027, 60.4721) projected
  line L1435 (-88.2027, 60.4721) -> (-88.1951, 60.438) projected
  line L1436 (-88.1951, 60.438) -> (-88.1882, 60.4038) projected
  line L1437 (-88.1882, 60.4038) -> (-88.1818, 60.3695) projected
  line L1438 (-88.1818, 60.3695) -> (-88.176, 60.3351) projected
  line L1439 (-88.176, 60.3351) -> (-88.1709, 60.3005) projected
  line L1440 (-88.1709, 60.3005) -> (-88.1663, 60.2659) projected
  line L1441 (-88.1663, 60.2659) -> (-88.1624, 60.2313) projected
  line L1442 (-88.1624, 60.2313) -> (-88.159, 60.1965) projected
  line L1443 (-88.159, 60.1965) -> (-88.1563, 60.1617) projected
  point P0 (0, 0)
extrude "Extrusão2" cut sketch "Esboço3" against normal blind 10 contours L4 L5 L6 L7 L8 L9 L10 L11 L12 L13 L14 L15 L16 L17 L18 L19 L20 L21 L22 L23 L24 L25 L26 L27 L28 L29 L30 L31 L32 L33 L34 L35 L36 L37 L38 L39 L40 L41 L42 L43 L44 L45 L46 L47 L48 L49 L50 L51 L52 L53 L54 L55 L56 L57 L58 L59 L60 L61 L62 L63 L64 L65 L66 L67 L68 L69 L70 L71 L72 L73 L74 L75 L76 L77 L78 L79 L80 L81 L82 L83 L84 L85 L86 L87 L88 L89 L90 L91 L92 L93 L94 L95 L96 L97 L98 L99 L100 L101 L102 L103 L104 L105 L106 L107 L108 L109 L110 L111 L112 L113 L114 L115 L116 L117 L118 L119 L120 L121 L122 L123 L124 L125 L126 L127 L128 L129 L130 L131 L132 L133 L134 L135 L136 L137 L138 L139 L140 L141 L142 L143 L144 L145 L146 L147 L148 L149 L150 L151 L152 L153 L154 L155 L156 L157 L158 L159 L160 L161 L162 L163 L164 L165 L166 L167 L168 L169 L170 L171 L172 L173 L174 L175 L176 L177 L178 L179 L180 L181 L182 L183 L184 L185 L186 L187 L188 L189 L190 L191 L192 L193 L194 L195 L196 L197 L198 L199 L200 L201 L202 L203 L204 L205 L206 L207 L208 L209 L210 L211 L212 L213 L214 L215 L216 L217 L218 L219 L220 L221 L222 L223 L224 L225 L226 L227 L228 L229 L230 L231 L232 L233 L234 L235 L236 L237 L238 L239 L240 L241 L242 L243 L244 L245 L246 L247 L248 L249 L250 L251 L252 L253 L254 L255 L256 L257 L258 L259 L260 L261 L262 L263 L264 L265 L266 L267 L268 L269 L270 L271 L272 L273 L274 L275 L276 L277 L278 L279 L280 L281 L282 L283 L284 L285 L286 L287 L288 L289 L290 L291 L292 L293 L294 L295 L296 L297 L298 L299 L300 L301 L302 L303 L304 L305 L306 L307 L308 L309 L310 L311 L312 L313 L314 L315 L316 L317 L318 L319 L320 L321 L322 L323 L324 L325 L326 L327 L328 L329 L330 L331 L332 L333 L334 L335 L336 L337 L338 L339 L340 L341 L342 L343 L344 L345 L346 L347 L348 L349 L350 L351 L352 L353 L354 L355 L356 L357 L358 L359 L360 L361 L362 L363 | L364 L365 L366 L367 L368 L369 L370 L371 L372 L373 L374 L375 L376 L377 L378 L379 L380 L381 L382 L383 L384 L385 L386 L387 L388 L389 L390 L391 L392 L393 L394 L395 L396 L397 L398 L399 L400 L401 L402 L403 L404 L405 L406 L407 L408 L409 L410 L411 L412 L413 L414 L415 L416 L417 L418 L419 L420 L421 L422 L423 L424 L425 L426 L427 L428 L429 L430 L431 L432 L433 L434 L435 L436 L437 L438 L439 L440 L441 L442 L443 L444 L445 L446 L447 L448 L449 L450 L451 L452 L453 L454 L455 L456 L457 L458 L459 L460 L461 L462 L463 L464 L465 L466 L467 L468 L469 L470 L471 L472 L473 L474 L475 L476 L477 L478 L479 L480 L481 L482 L483 L484 L485 L486 L487 L488 L489 L490 L491 L492 L493 L494 L495 L496 L497 L498 L499 L500 L501 L502 L503 L504 L505 L506 L507 L508 L509 L510 L511 L512 L513 L514 L515 L516 L517 L518 L519 L520 L521 L522 L523 L524 L525 L526 L527 L528 L529 L530 L531 L532 L533 L534 L535 L536 L537 L538 L539 L540 L541 L542 L543 L544 L545 L546 L547 L548 L549 L550 L551 L552 L553 L554 L555 L556 L557 L558 L559 L560 L561 L562 L563 L564 L565 L566 L567 L568 L569 L570 L571 L572 L573 L574 L575 L576 L577 L578 L579 L580 L581 L582 L583 L584 L585 L586 L587 L588 L589 L590 L591 L592 L593 L594 L595 L596 L597 L598 L599 L600 L601 L602 L603 L604 L605 L606 L607 L608 L609 L610 L611 L612 L613 L614 L615 L616 L617 L618 L619 L620 L621 L622 L623 L624 L625 L626 L627 L628 L629 L630 L631 L632 L633 L634 L635 L636 L637 L638 L639 L640 L641 L642 L643 L644 L645 L646 L647 L648 L649 L650 L651 L652 L653 L654 L655 L656 L657 L658 L659 L660 L661 L662 L663 L664 L665 L666 L667 L668 L669 L670 L671 L672 L673 L674 L675 L676 L677 L678 L679 L680 L681 L682 L683 L684 L685 L686 L687 L688 L689 L690 L691 L692 L693 L694 L695 L696 L697 L698 L699 L700 L701 L702 L703 L704 L705 L706 L707 L708 L709 L710 L711 L712 L713 L714 L715 L716 L717 L718 L719 L720 L721 L722 L723 | L724 L725 L726 L727 L728 L729 L730 L731 L732 L733 L734 L735 L736 L737 L738 L739 L740 L741 L742 L743 L744 L745 L746 L747 L748 L749 L750 L751 L752 L753 L754 L755 L756 L757 L758 L759 L760 L761 L762 L763 L764 L765 L766 L767 L768 L769 L770 L771 L772 L773 L774 L775 L776 L777 L778 L779 L780 L781 L782 L783 L784 L785 L786 L787 L788 L789 L790 L791 L792 L793 L794 L795 L796 L797 L798 L799 L800 L801 L802 L803 L804 L805 L806 L807 L808 L809 L810 L811 L812 L813 L814 L815 L816 L817 L818 L819 L820 L821 L822 L823 L824 L825 L826 L827 L828 L829 L830 L831 L832 L833 L834 L835 L836 L837 L838 L839 L840 L841 L842 L843 L844 L845 L846 L847 L848 L849 L850 L851 L852 L853 L854 L855 L856 L857 L858 L859 L860 L861 L862 L863 L864 L865 L866 L867 L868 L869 L870 L871 L872 L873 L874 L875 L876 L877 L878 L879 L880 L881 L882 L883 L884 L885 L886 L887 L888 L889 L890 L891 L892 L893 L894 L895 L896 L897 L898 L899 L900 L901 L902 L903 L904 L905 L906 L907 L908 L909 L910 L911 L912 L913 L914 L915 L916 L917 L918 L919 L920 L921 L922 L923 L924 L925 L926 L927 L928 L929 L930 L931 L932 L933 L934 L935 L936 L937 L938 L939 L940 L941 L942 L943 L944 L945 L946 L947 L948 L949 L950 L951 L952 L953 L954 L955 L956 L957 L958 L959 L960 L961 L962 L963 L964 L965 L966 L967 L968 L969 L970 L971 L972 L973 L974 L975 L976 L977 L978 L979 L980 L981 L982 L983 L984 L985 L986 L987 L988 L989 L990 L991 L992 L993 L994 L995 L996 L997 L998 L999 L1000 L1001 L1002 L1003 L1004 L1005 L1006 L1007 L1008 L1009 L1010 L1011 L1012 L1013 L1014 L1015 L1016 L1017 L1018 L1019 L1020 L1021 L1022 L1023 L1024 L1025 L1026 L1027 L1028 L1029 L1030 L1031 L1032 L1033 L1034 L1035 L1036 L1037 L1038 L1039 L1040 L1041 L1042 L1043 L1044 L1045 L1046 L1047 L1048 L1049 L1050 L1051 L1052 L1053 L1054 L1055 L1056 L1057 L1058 L1059 L1060 L1061 L1062 L1063 L1064 L1065 L1066 L1067 L1068 L1069 L1070 L1071 L1072 L1073 L1074 L1075 L1076 L1077 L1078 L1079 L1080 L1081 L1082 L1083 | L1084 L1085 L1086 L1087 L1088 L1089 L1090 L1091 L1092 L1093 L1094 L1095 L1096 L1097 L1098 L1099 L1100 L1101 L1102 L1103 L1104 L1105 L1106 L1107 L1108 L1109 L1110 L1111 L1112 L1113 L1114 L1115 L1116 L1117 L1118 L1119 L1120 L1121 L1122 L1123 L1124 L1125 L1126 L1127 L1128 L1129 L1130 L1131 L1132 L1133 L1134 L1135 L1136 L1137 L1138 L1139 L1140 L1141 L1142 L1143 L1144 L1145 L1146 L1147 L1148 L1149 L1150 L1151 L1152 L1153 L1154 L1155 L1156 L1157 L1158 L1159 L1160 L1161 L1162 L1163 L1164 L1165 L1166 L1167 L1168 L1169 L1170 L1171 L1172 L1173 L1174 L1175 L1176 L1177 L1178 L1179 L1180 L1181 L1182 L1183 L1184 L1185 L1186 L1187 L1188 L1189 L1190 L1191 L1192 L1193 L1194 L1195 L1196 L1197 L1198 L1199 L1200 L1201 L1202 L1203 L1204 L1205 L1206 L1207 L1208 L1209 L1210 L1211 L1212 L1213 L1214 L1215 L1216 L1217 L1218 L1219 L1220 L1221 L1222 L1223 L1224 L1225 L1226 L1227 L1228 L1229 L1230 L1231 L1232 L1233 L1234 L1235 L1236 L1237 L1238 L1239 L1240 L1241 L1242 L1243 L1244 L1245 L1246 L1247 L1248 L1249 L1250 L1251 L1252 L1253 L1254 L1255 L1256 L1257 L1258 L1259 L1260 L1261 L1262 L1263 L1264 L1265 L1266 L1267 L1268 L1269 L1270 L1271 L1272 L1273 L1274 L1275 L1276 L1277 L1278 L1279 L1280 L1281 L1282 L1283 L1284 L1285 L1286 L1287 L1288 L1289 L1290 L1291 L1292 L1293 L1294 L1295 L1296 L1297 L1298 L1299 L1300 L1301 L1302 L1303 L1304 L1305 L1306 L1307 L1308 L1309 L1310 L1311 L1312 L1313 L1314 L1315 L1316 L1317 L1318 L1319 L1320 L1321 L1322 L1323 L1324 L1325 L1326 L1327 L1328 L1329 L1330 L1331 L1332 L1333 L1334 L1335 L1336 L1337 L1338 L1339 L1340 L1341 L1342 L1343 L1344 L1345 L1346 L1347 L1348 L1349 L1350 L1351 L1352 L1353 L1354 L1355 L1356 L1357 L1358 L1359 L1360 L1361 L1362 L1363 L1364 L1365 L1366 L1367 L1368 L1369 L1370 L1371 L1372 L1373 L1374 L1375 L1376 L1377 L1378 L1379 L1380 L1381 L1382 L1383 L1384 L1385 L1386 L1387 L1388 L1389 L1390 L1391 L1392 L1393 L1394 L1395 L1396 L1397 L1398 L1399 L1400 L1401 L1402 L1403 L1404 L1405 L1406 L1407 L1408 L1409 L1410 L1411 L1412 L1413 L1414 L1415 L1416 L1417 L1418 L1419 L1420 L1421 L1422 L1423 L1424 L1425 L1426 L1427 L1428 L1429 L1430 L1431 L1432 L1433 L1434 L1435 L1436 L1437 L1438 L1439 L1440 L1441 L1442 L1443